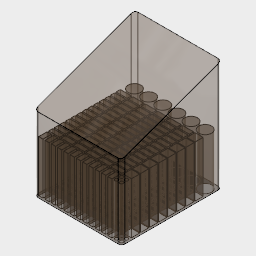
6_col_block (Autodesk Fusion 360 design; units mm, degrees)
Autodesk Fusion 360 part; units mm, degrees
sketch "Sketch1" plane through (0, 0, 0) normal (0, 1, 0) x (1, 0, 0)
  line L0 (51.1, 58.7) -> (-51.1, 58.7)
  line L1 (-51.1, 58.7) -> (-51.1, -58.7)
  line L2 (-51.1, -58.7) -> (51.1, -58.7)
  line L3 (51.1, -58.7) -> (51.1, 58.7)
  line L4 (51.1, 58.7) -> (-51.1, -58.7) construction
  line L5 (-51.1, 58.7) -> (51.1, -58.7) construction
  line L6 (-43.6, -56.2) -> (-48.6, -56.2)
  line L7 (-48.6, -56.2) -> (-48.6, -46.2)
  line L8 (-48.6, -46.2) -> (-43.6, -46.2)
  line L9 (-43.6, -46.2) -> (-43.6, -56.2)
  line L10 (-48.6, -44.6) -> (-35.6, -44.6)
  line L11 (-35.6, -44.6) -> (-35.6, -39.6)
  line L12 (-35.6, -39.6) -> (-48.6, -39.6)
  line L13 (-48.6, -39.6) -> (-48.6, -44.6)
  circle A0 centre (-41.1, 48.7) radius 7.5
  circle A1 centre (46.6, -54.2) radius 2
  line L14 (48.6, -44.6) -> (39, -44.6)
  line L15 (39, -44.6) -> (39, -35)
  line L16 (39, -35) -> (48.6, -35)
  line L17 (48.6, -35) -> (48.6, -44.6)
  dimension "d1" = 102.2
  dimension "d2" = 117.4
  dimension "d3" = 5
  dimension "d4" = 10
  dimension "d5" = 2.5
  dimension "d6" = 2.5
  dimension "d7" = 13
  dimension "d8" = 5
  dimension "d9" = 1.6
  dimension "d10" = 15
  dimension "d11" = 10
  dimension "d12" = 10
  dimension "d13" = 4
  dimension "d14" = 4.5
  dimension "d15" = 4.5
  dimension "d16" = 9.6
  dimension "d17" = 9.6
  dimension "d18" = 2.5
  dimension "d19" = 9.6
  measures "d1" distance of L1.end L2.end
  measures "d2" distance of L0.start L2.end
  measures "d3" distance of L6.start L6.end
  measures "d4" distance of L6.start L8.end
  measures "d5" distance of L2 L6
  measures "d6" distance of L1 L7
  measures "d7" distance of L11.end L12.end
  measures "d8" distance of L10.end L11.end
  measures "d9" distance of L8 L10
  measures "d10" diameter of A0
  measures "d11" distance of L0 A0.centre
  measures "d12" distance of L1 A0.centre
  measures "d13" diameter of A1
  measures "d14" distance of L3 A1.centre
  measures "d15" distance of L2 A1.centre
  measures "d16" distance of L14.start L16.end
  measures "d17" distance of L14.start L14.end
  measures "d18" distance of L3 L17
  measures "d19" distance of A1.centre L14
extrude "Extrude1" add sketch "Sketch1" along normal blind 130 contours L0 L1 L2 L3 | L6 L7 L8 L9 | L10 L11 L12 L13 | A0 | A1 | L14 L15 L16 L17
extrude "Extrude2" cut sketch "Sketch1" along normal blind 60 contours L6 L7 L8 L9
extrude "Extrude3" cut sketch "Sketch1" along normal blind 60 contours L10 L11 L12 L13
extrude "Extrude4" cut sketch "Sketch1" along normal blind 60 contours L14 L15 L16 L17
extrude "Extrude5" cut sketch "Sketch1" along normal blind 60 contours A1
extrude "Extrude6" cut sketch "Sketch1" along normal blind 60 contours A0
pattern_linear "R-Pattern1" count 12 spacing 7.3636 along (1, 0, 0) of "Extrude2"
pattern_linear "R-Pattern2" count 6 spacing 14.6 along (1, 0, 0) count 13 spacing 6.6 along (0, 0, -1) of "Extrude3"
pattern_linear "R-Pattern3" count 1 spacing 0 along (-1, 0, 0) count 8 spacing 10.6571 along (0, 0, -1) of "Extrude4"
pattern_linear "R-Pattern4" count 2 spacing 5.6 along (-1, 0, 0) count 2 spacing 5.6 along (0, 0, -1) of "Extrude5"
pattern_linear "R-Pattern5" count 6 spacing 16.6 along (1, 0, 0) of "Extrude6"
sketch "Sketch2" plane through (-51.1, 0, 0) normal (-1, 0, 0) x (0, 0, 1)
  line L0 (-58.7, 0) -> (58.7, 0)
  line L1 (58.7, 0) -> (58.7, 130)
  line L2 (58.7, 130) -> (-58.7, 130)
  line L3 (-58.7, 130) -> (-58.7, 0)
  line L4 (-58.7, 130) -> (58.7, 87.2699)
  dimension "d52" = 20
  measures "d52" angle of L2 L4
extrude "Extrude7" cut sketch "Sketch2" against normal through all and the other way blind 0 contours L1 L2 L4
fillet "Fillet1" radius 4 4 edges at (-51.1, 43.6349, 58.7) (51.1, 43.6349, 58.7) (-51.1, 65, -58.7) (51.1, 65, -58.7)
equation "d2 = 109.9 mm + 7.5 mm"
